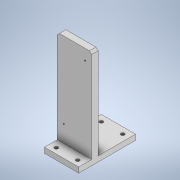
# Autodesk Inventor part: L periscope
Saved by Autodesk Inventor 2020 (Build 240168000, 168)
## iProperties
Created: 2020-10-30
Part Number: L periscope
Material: Generic
Document SubType Name: Modeling
Designer: Austin
Density: 1 g/cm^3
Appearance: Default
Author: Austin
Autodesk Inventor part; units mm, degrees
ref_plane "YZ Plane" through (0, 0, 0) normal (1, 0, 0) x (0, 1, 0)
ref_plane "XZ Plane" through (0, 0, 0) normal (0, 1, 0) x (-1, 0, 0)
ref_plane "XY Plane" through (0, 0, 0) normal (0, 0, 1) x (1, 0, 0)
sketch "Sketch1" plane through (0, 0, 0) normal (0, 1, 0) x (-1, 0, 0)
  line L0 (16, 3) -> (-16, 3)
  line L1 (-16, 3) -> (-16, -3)
  line L2 (-16, -3) -> (16, -3)
  line L3 (16, -3) -> (16, 3)
  line L4 (16, 3) -> (-16, -3) construction
  line L5 (-16, 3) -> (16, -3) construction
  point P0 (0, 0)
  dimension "POST_THICKNESS" = 6
  dimension "POST_WIDTH" = 32
  constraints: 12 end point, 2 midpoint, 2 parallel, 1 horizontal, 1 perpendicular
  measures "POST_THICKNESS" distance of L2.end L0.start
  measures "POST_WIDTH" distance of L0.start L0.end
extrude "Extrusion1" add sketch "Sketch1" along normal blind 73.912
sketch "Sketch5" plane through (16, 73.912, -3) normal (0, 0, -1) x (-1, 0, 0)
  line L0 (0, 0) -> (32, 0) projected
  line L1 (16.088, 0) -> (0, -16.088)
  line L2 (0, -73.912) -> (0, 0) projected
  circle A0 centre (6.088, -10) radius 1.75
  circle A1 centre (9.6235, -6.4645) radius 1
  circle A2 centre (2.5525, -13.5355) radius 1
  line L3 (32.1913, -64.8447) -> (19.6606, -77.3754)
  circle A3 centre (29.4475, -67.5885) radius 1
  circle A4 centre (22.3765, -74.6595) radius 1
  line L4 (32, -73.912) -> (32, 0) projected
  circle A5 centre (25.912, -71.124) radius 1.75
  line L5 (0, -73.912) -> (32, -73.912) projected
  point P0 (16, -73.912)
  point P1 (0, -58)
  point P2 (32, -58)
  dimension "d33" = 45
  dimension "d35" = 0
  dimension "d36" = 5
  dimension "d37" = 5
  dimension "d38" = 45
  dimension "d39" = 9.9999
  dimension "d42" = 0
  dimension "d43" = 5
  dimension "d44" = 2
  dimension "d45" = 2
  dimension "d46" = 2
  dimension "d47" = 2
  dimension "BOTTOM_MIRROR_HOLE" = 2.788
  dimension "TOP_MIRROR_HOLE" = 63.912
  dimension "d90" = 9.912
  dimension "d91" = 9.912
  dimension "d92" = 3.5
  dimension "d93" = 3.5
  constraints: 6 centre point, 6 point on line, 4 end point, 1 other
  measures "d33" angle of L1 L2
  measures "d35" distance from line of L1 A0.centre
  measures "d36" distance of A0.centre A1.centre
  measures "d37" distance of A2.centre A0.centre
  measures "d38" angle to the sketch x axis of L3
  measures "d39" distance of A4.centre A3.centre
  measures "d42" distance from line of L3 A5.centre
  measures "d43" distance of A5.centre A3.centre
  measures "d44" diameter of A2
  measures "d45" diameter of A1
  measures "d46" diameter of A4
  measures "d47" diameter of A3
  measures "BOTTOM_MIRROR_HOLE" distance from line of L5 A5.centre
  measures "TOP_MIRROR_HOLE" distance from line of L5 A0.centre
  measures "d90" horizontal distance of point (16, -73.912) A0.centre
  measures "d91" horizontal distance of point (16, -73.912) A5.centre
  measures "d92" diameter of A0
  measures "d93" diameter of A5
extrude "Extrusion3" cut sketch "Sketch5" against normal blind 3 contours A1 L1 | L1 A1 | A2 L1 | L1 A2 | L5 A4 L3 | A4 L5 | A3 L3 | L3 A3 | L3 A4 picked at (22.0928, -74.8345)
sketch "Sketch6" plane through (16, 0, -3) normal (0, 0, -1) x (-1, 0, 0)
  line L0 (0, 0) -> (0, 73.912) projected
  line L1 (0, 0) -> (32, 0) projected
  line L2 (0, 2) -> (32, 2)
  line L3 (32, 2) -> (32, 0)
  line L4 (32, 0) -> (0, 0)
  line L5 (0, 0) -> (0, 2)
  point P0 (16, 0)
  dimension "BASE_HEIGHT" = 2
  constraints: 8 end point, 2 parallel, 1 horizontal, 1 perpendicular, 1 point on line
  measures "BASE_HEIGHT" distance between parallel lines of L1 L2
extrude "Extrusion4" [suppressed]
sketch "Sketch7" plane through (-16, 2, -3) normal (0, 1, 0) x (1, 0, 0)
  line L0 (0, 35) -> (32, 35) projected
  line L1 (0, 0) -> (0, 35) projected
  line L2 (32, 0) -> (32, 35) projected
  point P0 (16, -3)
  point P1 (26, 29)
  point P2 (6, 29)
  dimension "d60" = 6
  dimension "d61" = 6
  dimension "d62" = 6
  dimension "d63" = 0
  measures "d60" distance from line of L0 point (6, 29)
  measures "d61" distance from line of L1 point (6, 29)
  measures "d62" distance from line of L2 point (26, 29)
  measures "d63" vertical distance of point (6, 29) point (26, 29)
hole "Hole3" [suppressed]
sketch "Sketch8" plane through (16, 73.912, -3) normal (0, 0, -1) x (-1, 0, 0)
  line L0 (0, 0) -> (32, 0)
  line L1 (12.088, 0) -> (0, -12.088)
  line L2 (0, -60) -> (0, 0)
  circle A0 centre (6.088, -6) radius 1.651
  circle A1 centre (9.6235, -2.4645) radius 1
  circle A2 centre (2.5525, -9.5355) radius 1
  line L3 (32.1913, -28.7207) -> (19.6606, -41.2514)
  circle A3 centre (29.4475, -31.4645) radius 1
  circle A4 centre (22.3765, -38.5355) radius 1
  line L4 (32, -60) -> (32, 0)
  circle A5 centre (25.912, -35) radius 1.651
  point P0 (16, -73.912)
  point P1 (16, -60)
  point P2 (0, -58)
  point P3 (32, -58)
  dimension "d64" = 45
  dimension "d65" = 0
  dimension "d66" = 5
  dimension "d67" = 5
  dimension "d68" = 45
  dimension "d69" = 9.9999
  dimension "d70" = 0
  dimension "d71" = 5
  dimension "d72" = 2
  dimension "d73" = 2
  dimension "d74" = 2
  dimension "d75" = 2
  constraints: 8 end point, 6 centre point, 6 point on line, 3 other
  measures "d64" angle of L1 L2
  measures "d65" distance from line of L1 A0.centre
  measures "d66" distance of A0.centre A1.centre
  measures "d67" distance of A2.centre A0.centre
  measures "d68" angle to the sketch x axis of L3
  measures "d69" distance of A4.centre A3.centre
  measures "d70" distance from line of L3 A5.centre
  measures "d71" distance of A5.centre A3.centre
  measures "d72" diameter of A2
  measures "d73" diameter of A1
  measures "d74" diameter of A4
  measures "d75" diameter of A3
hole "Hole4" [suppressed]
chamfer "Chamfer1" distance 2 angle 45 2 edges at (-16, 73.912, 0) (16, 73.912, 0)
hole "Hole5" at (9.912, 63.912, -3) at (-9.912, 2.788, -3) direction (0, 0, 1) diameter 4.496 depth 5 tip angle 118 clearance for "Flat Head Machine Screw (82)" size "#8" standard "Ansi Unified Screw Threads"
sketch "Sketch10" plane through (0, 0, 0) normal (0, -1, 0) x (1, 0, 0)
  line L0 (14, 3) -> (16, 3) projected
  line L1 (-14, -3) -> (-16, -3) projected
  line L2 (16, 3) -> (-16, 3)
  line L3 (-16, 3) -> (-16, -3)
  line L4 (-16, -3) -> (16, -3)
  line L5 (16, -3) -> (16, 3)
  point P0 (0, 0)
  constraints: 8 end point, 2 parallel, 1 horizontal, 1 perpendicular
extrude "Extrusion6" add sketch "Sketch10" along normal blind 18
sketch "Sketch11" plane through (0, -18, 0) normal (0, -1, 0) x (1, 0, 0)
  line L0 (16, 25) -> (-16, 25)
  line L1 (-16, 25) -> (-16, -38)
  line L2 (-16, -38) -> (16, -38)
  line L3 (16, -38) -> (16, 25)
  line L4 (-16, 25) -> (16, 25)
  line L5 (16, 25) -> (16, 15)
  line L6 (16, 15) -> (-16, 15)
  line L7 (-16, 15) -> (-16, 25)
  line L8 (16, -3) -> (-16, -3)
  point P0 (0, 0)
  point P1 (-16, 15)
  dimension "d107" = 32
  dimension "d124" = 10
  dimension "d125" = 35
  constraints: 18 end point, 4 parallel, 3 horizontal, 2 perpendicular, 1 point on line
  measures "d107" distance of L0.start L0.end
  measures "d124" distance between parallel lines of L6 L0
  measures "d125" distance between parallel lines of L2 L8
extrude "Extrusion7" add sketch "Sketch11" against normal blind 5 contours L3 L8 L1 L6 | L3 L2 L1 L8
sketch "Sketch12" plane through (0, -13, 0) normal (0, 1, 0) x (1, 0, 0)
  point P0 (0, 0)
  point P1 (-10, 32)
  point P2 (10, 32)
  point P3 (-10, -10)
  point P4 (10, -10)
  dimension "d116" = 10
  dimension "d117" = 10
  dimension "d118" = 32
  dimension "d119" = 32
  dimension "d120" = 10
  dimension "d121" = 10
  dimension "d122" = 20
  dimension "d123" = 10
  measures "d116" horizontal distance of point (0, 0) point (-10, 32)
  measures "d117" horizontal distance of point (10, 32) point (0, 0)
  measures "d118" vertical distance of point (0, 0) point (-10, 32)
  measures "d119" vertical distance of point (10, 32) point (0, 0)
  measures "d120" horizontal distance of point (0, 0) point (-10, -10)
  measures "d121" horizontal distance of point (10, -10) point (0, 0)
  measures "d122" distance of point (10, -10) point (-10, -10)
  measures "d123" horizontal distance of point (0, 0) point (-10, -10)
hole "Hole6" at (-10, -13, -32) at (10, -13, -32) at (-10, -13, 10) at (10, -13, 10) direction (0, -1, 0) diameter 3.302 depth 8 thread size "8-32 UNC" class "2B" standard "ANSI Unified Screw Threads"
sketch "Sketch14" plane through (0, -13, 0) normal (0, 1, 0) x (1, 0, 0)
  line L0 (-16, -15) -> (-16, 38) projected
  line L1 (-16, 27) -> (-12.9595, 27)
  line L2 (-10.9595, 25) -> (-10.9595, 23)
  line L3 (-12.9595, 21) -> (-16, 21)
  line L4 (-16, 21) -> (-16, 27)
  line L5 (14, 3) -> (-14, 3) projected
  arc A0 (-12.9595, 21) -> (-10.9595, 23) centre (-12.9595, 23) ccw
  arc A1 (-10.9595, 25) -> (-12.9595, 27) centre (-12.9595, 25) ccw
  point P0 (0, 0)
  point P1 (-10.9595, 21)
  point P2 (-10.9595, 27)
  dimension "d127" = 6
  dimension "d128" = 18
  dimension "d131" = 2
  constraints: 8 end point, 5 point on line, 4 point on circle, 4 tangent, 2 centre point, 2 parallel, 1 equal radius, 1 horizontal, 1 perpendicular
  measures "d127" distance between parallel lines of L1 L3
  measures "d128" distance between parallel lines of L5 L3
  measures "d131" radius of A0
extrude "Extrusion8" cut sketch "Sketch14" against normal blind 10
extrude "Extrusion9" cut sketch "Sketch5" against normal blind 3 contours L5 A4 L3 | A4 L5 | L3 A4 picked at (22.0928, -74.8345)
equation "\"BOTTOM_MIRROR_HOLE\" = GROUND_BEAM_HEIGHT - POLARIS_HOLE_TO_MIRROR_HEIGHT"
equation "\"TOP_MIRROR_HOLE\" = LASER_BEAM_HEIGHT + POLARIS_HOLE_TO_MIRROR_HEIGHT"
equation "\"d90\" = POLARIS_HOLE_TO_MIRROR_HEIGHT"
equation "\"d91\" = POLARIS_HOLE_TO_MIRROR_HEIGHT"
equation "\"WING_SIZE\" = 8"
equation "\"POLARIS_HOLE_TO_MIRROR_HEIGHT\" = 9.912"
equation "\"GROUND_BEAM_HEIGHT\" = 12.7"
equation "\"LASER_BEAM_HEIGHT\" = 54"
body "Solid1"
